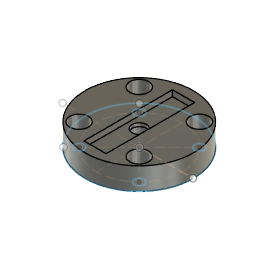
Acoplador_CelulaDeCarga_Uniaxial (Autodesk Fusion 360 design; units mm, degrees)
Autodesk Fusion 360 part; units mm, degrees
note: some values were not read from the file. Chosen so that the rebuilt part matches the saved one: that a step has no effect.
sketch "Esboço41" plane through (0, 0, 0) normal (0, 0, 1) x (1, 0, 0)
  line L0 (200, 0) -> (222.4506, -22.4506) construction
  line L1 (200, 0) -> (231.75, 0) construction
  line L2 (200, 25) -> (200, -25) construction
  line L3 (200, 0) -> (177.7261, 22.2739) construction
  line L4 (200, 0) -> (155, 0) construction
  circle A0 centre (182.3223, 17.6777) radius 2.75
  line L5 (200, 0) -> (177.7261, -22.2739) construction
  circle A1 centre (217.6777, 17.6777) radius 2.75
  line L6 (200, 0) -> (231.5, 0) construction
  circle A2 centre (200, 0) radius 31.75
  line L7 (200, 0) -> (231.5, 0) construction
  line L8 (200, 0) -> (222.4506, 22.4506) construction
  circle A3 centre (217.6777, -17.6777) radius 2.75
  circle A4 centre (182.3223, -17.6777) radius 2.75
  circle A5 centre (200, 0) radius 25 construction
  point P0 (200, 0)
  point P1 (200, 0)
  dimension "d222" = 63.5
  dimension "d223" = 45
  dimension "d224" = 135
  dimension "d225" = 135
  dimension "d226" = 50
  dimension "d227" = 5.5
  dimension "d228" = 5.5
  dimension "d229" = 5.5
  dimension "d230" = 5.5
  constraint coincident P1 P0
  constraint horizontal L1
  constraint coincident L8.end A2
  constraint coincident L1.end A2
  constraint horizontal L7
  constraint horizontal L6
  constraint coincident P0 L0.start
  constraint coincident L0.end A2
  constraint perpendicular L0 L8
  constraint concentric A2 A5
  constraint coincident A0.centre A5
  constraint coincident A0.centre L3
  constraint coincident A1.centre L8
  constraint coincident A1.centre A5
  constraint coincident A4.centre A5
  constraint coincident A4.centre L5
  constraint coincident A3.centre L0
  constraint coincident A3.centre A5
  constraint horizontal L4
  constraint coincident L2.start A5
  constraint coincident L2.end A5
  constraint perpendicular L2 L4
  measures "d222" diameter of A2
  measures "d223" angle of L1 L8
  measures "d224" angle of L3 L7
  measures "d225" angle of L5 L6
  measures "d226" diameter of A5
  measures "d227" diameter of A0
  measures "d228" diameter of A1
  measures "d229" diameter of A4
  measures "d230" diameter of A3
extrude "Extrusão51" [no effect]
extrude "Extrusão59" add sketch "Esboço41" along normal blind 13
sketch "Esboço52" plane through (0, 0, 13) normal (0, 0, 1) x (1, 0, 0)
  line L0 (193.5, -26) -> (206.5, -26)
  line L1 (206.5, -26) -> (206.5, 26)
  line L2 (206.5, 26) -> (193.5, 26)
  line L3 (193.5, 26) -> (193.5, -26)
  circle A0 centre (182.3223, -17.6777) radius 2.75
  circle A1 centre (182.3223, 17.6777) radius 2.75
  circle A2 centre (217.6777, 17.6777) radius 2.75
  circle A3 centre (217.6777, -17.6777) radius 2.75
  circle A4 centre (200, 0) radius 31.75
  dimension "d292" = 13
  dimension "d293" = 52
  constraint horizontal L0
  constraint vertical L1
  constraint horizontal L2
  constraint vertical L3
  measures "d292" distance of L0.start L0.end
  measures "d293" distance of L0.start L2.end
extrude "Extrusão60" cut sketch "Esboço52" against normal blind 5 contours L0 L1 L2 L3
sketch "Esboço53" plane through (0, 0, 13) normal (0, 0, 1) x (-1, 0, 0)
  line L0 (-206.5, 26) -> (-193.5, 26)
  line L1 (-193.5, 26) -> (-193.5, -26)
  line L2 (-193.5, -26) -> (-206.5, -26)
  line L3 (-206.5, -26) -> (-206.5, 26)
  circle A0 centre (-182.3223, 17.6777) radius 2.75
  circle A1 centre (-182.3223, -17.6777) radius 2.75
  circle A2 centre (-217.6777, -17.6777) radius 2.75
  circle A3 centre (-217.6777, 17.6777) radius 2.75
  circle A4 centre (-200, 0) radius 31.75
  circle A5 centre (-217.6777, 17.6777) radius 5.5
  circle A6 centre (-182.3223, 17.6777) radius 5.5
  circle A7 centre (-217.6777, -17.6777) radius 5.5
  circle A8 centre (-182.3223, -17.6777) radius 5.5
  dimension "d296" = 11
  dimension "d297" = 11
  dimension "d298" = 11
  dimension "d299" = 11
  constraint concentric A3 A5
  constraint concentric A0 A6
  constraint concentric A2 A7
  constraint concentric A1 A8
  measures "d296" diameter of A5
  measures "d297" diameter of A6
  measures "d298" diameter of A7
  measures "d299" diameter of A8
extrude "Extrusão61" cut sketch "Esboço53" against normal blind 11 contours A5 | A6 | A7 | A8
sketch "Esboço54" plane through (0, 0, 0) normal (0, 0, 1) x (1, 0, 0)
  circle A0 centre (200, 0) radius 8.5
  dimension "d302" = 17
  measures "d302" diameter of A0
extrude "Extrusão62" add 1 faces at (197.8333, -8.6667, 8) along direction (0, 0, 1) blind 1.5
extrude "Extrusão63" cut sketch "Esboço54" along normal blind 7.5
sketch "Esboço56" plane through (0, 0, 0) normal (0, 0, 1) x (1, 0, 0)
  circle A0 centre (200, 0) radius 4.25
  dimension "d307" = 8.5
  measures "d307" diameter of A0
extrude "Extrusão64" cut sketch "Esboço56" along normal blind 20
